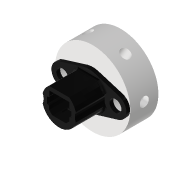
# Autodesk Inventor part: 00_toslink_launcher_v3
Saved by Autodesk Inventor 2022 (Build 260153000, 153)
## iProperties
Created: 2022-08-14
Part Number: 00_toslink_launcher_v3
Material: Generic
Document SubType Name: Modeling
Designer: diederichbenedict
Density: 1 g/cm^3
Appearance: Default
Author: diederichbenedict
Autodesk Inventor part; units mm, degrees
ref_plane "YZ Plane" through (0, 0, 0) normal (1, 0, 0) x (0, 1, 0)
ref_plane "XZ Plane" through (0, 0, 0) normal (0, 1, 0) x (-1, 0, 0)
ref_plane "XY Plane" through (0, 0, 0) normal (0, 0, 1) x (1, 0, 0)
sketch "Skizze1" plane through (-3.3485, 5.2472, 0) normal (0, 0, -1) x (-1, 0, 0)
  arc A0 (-5.1663, -7.5068) -> (-0.7991, -6.6295) centre (-3.3485, -5.2472) ccw
  line L0 (-0.3985, -7.0082) -> (-3.2985, -8.6825)
  line L1 (-0.3485, -3.5729) -> (-0.3485, -6.9216)
  line L2 (-3.2985, -1.812) -> (-0.3985, -3.4863)
  arc A1 (-0.4995, -5.7887) -> (-5.5773, -3.3919) centre (-3.3485, -5.2472) ccw
  line L3 (-6.2985, -3.4863) -> (-3.3985, -1.812)
  line L4 (-6.3485, -6.9216) -> (-6.3485, -3.5729)
  line L5 (-0.3485, -6.9793) -> (-3.3485, -8.7113)
  line L6 (-3.3485, -8.7113) -> (-6.3485, -6.9793)
  line L7 (-6.3485, -6.9793) -> (-6.3485, -3.5152)
  line L8 (-6.3485, -3.5152) -> (-3.3485, -1.7831)
  line L9 (-3.3485, -1.7831) -> (-0.3485, -3.5152)
  line L10 (-0.3485, -3.5152) -> (-0.3485, -6.9793)
  line L11 (0.1515, -3.2265) -> (0.1515, -7.268)
  line L12 (0.1515, -7.268) -> (-3.3485, -9.2887)
  line L13 (-3.3485, -9.2887) -> (-6.8485, -7.268)
  line L14 (-6.8485, -7.268) -> (-6.8485, -3.2265)
  line L15 (-6.8485, -3.2265) -> (-3.3485, -1.2058)
  line L16 (-3.3485, -1.2058) -> (0.1515, -3.2265)
  circle A2 centre (-3.3485, -5.2472) radius 12.0305
  circle A3 centre (5.1515, -5.2472) radius 1.9
  circle A4 centre (-11.8485, -5.2472) radius 1.9
  point P0 (-3.3485, -5.2472)
extrude "Extrusion1" add sketch "Skizze1" along normal blind 9 contours A2
sketch "Skizze2" plane through (0, 4.0414, -9) normal (-0.5, -0.866, 0) x (0.866, -0.5, 0)
  line L0 (4.0415, 9) -> (4.0415, 0) projected
  line L1 (0, 9) -> (0, 0) projected
  circle A0 centre (2.1651, 4.5) radius 1.4
  point P0 (2.0207, 9)
  dimension "d3" = 2.8
  constraints: 1 centre point
  measures "d3" diameter of A0
extrude "Extrusion2" cut sketch "Skizze2" along normal through all both and the other way through all
pattern_circular "Runde Anordnung1" count 6 over 360 about axis through (0, 0, 0) along (0, 0, -1) of "Extrusion2"
